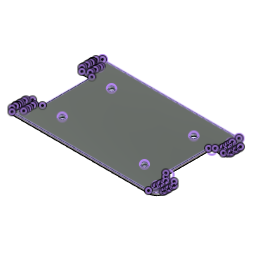
PCB Base (Autodesk Fusion 360 design; units mm, degrees)
Autodesk Fusion 360 part; units mm, degrees
note: some values were not read from the file. Set by a fixed rule: which sketch regions a step uses.
sketch "Sketch1" plane through (0, 0, 0) normal (0, 0, 1) x (1, 0, 0)
  line L0 (45, 27.5) -> (-45, 27.5)
  line L1 (-45, 27.5) -> (-45, -27.5)
  line L2 (-45, -27.5) -> (45, -27.5)
  line L3 (45, -27.5) -> (45, 27.5)
  line L4 (45, 27.5) -> (-45, -27.5) construction
  line L5 (-45, 27.5) -> (45, -27.5) construction
  dimension "d1" = 90
  dimension "d2" = 55
  constraint horizontal L0
  constraint perpendicular L0 L1
  constraint parallel L0 L2
  constraint parallel L1 L3
  constraint coincident L4 origin
  constraint coincident L5 origin
  measures "d1" distance of L1.end L2.end
  measures "d2" distance of L0.end L1.end
extrude "Extrude1" add sketch "Sketch1" along normal blind 1.6
fillet "Fillet1" radius 5 2 edges at (45, -27.5, 0.8) (45, 27.5, 0.8)
sketch "Sketch2" plane through (0, 0, 1.6) normal (0, 0, 1) x (-1, 0, 0)
  line L0 (45, -27.5) -> (45, 27.5)
  line L1 (45, 27.5) -> (-40, 27.5)
  arc A0 (-40, 27.5) -> (-45, 22.5) centre (-40, 22.5) ccw
  line L2 (-45, 22.5) -> (-45, -22.5)
  arc A1 (-45, -22.5) -> (-40, -27.5) centre (-40, -22.5) ccw
  line L3 (-40, -27.5) -> (45, -27.5)
  line L4 (25, 15) -> (-25, 15) construction
  line L5 (-25, 15) -> (-25, -15)
  line L6 (-25, -15) -> (25, -15) construction
  line L7 (25, -15) -> (25, 15)
  line L8 (25, 15) -> (-25, -15) construction
  line L9 (-25, 15) -> (25, -15) construction
  circle A2 centre (25, -15) radius 2
  circle A3 centre (25, 15) radius 1.8001
  circle A4 centre (-25, 15) radius 1.8646
  circle A5 centre (-25, -15) radius 2
  dimension "d10" = 50
  dimension "d11" = 30
  constraint horizontal L4
  constraint perpendicular L4 L5
  constraint parallel L4 L6
  constraint parallel L5 L7
  constraint coincident L8 origin
  constraint coincident L9 origin
  constraint coincident L6.end L7.start
  constraint coincident L4.start L7.end
  constraint coincident L4.end L5.start
  constraint coincident L5.end L6.start
  measures "d10" distance of L5.end L6.end
  measures "d11" distance of L4.end L5.end
extrude "Extrude2" cut sketch "Sketch2" against normal blind 4 contours A2 | A3 | A4 | A5
sketch "Sketch3" plane through (0, 0, 0) normal (0, 0, -1) x (1, 0, 0)
  circle A0 centre (25, -15) radius 2
  circle A1 centre (25, 15) radius 1.8646
  circle A2 centre (-25, -15) radius 2
  circle A3 centre (-25, 15) radius 1.8001
  line L0 (-45, -27.5) -> (40, -27.5)
  arc A4 (40, -27.5) -> (45, -22.5) centre (40, -22.5) ccw
  line L1 (45, -22.5) -> (45, 22.5)
  arc A5 (45, 22.5) -> (40, 27.5) centre (40, 22.5) ccw
  line L2 (40, 27.5) -> (-45, 27.5)
  line L3 (-45, 27.5) -> (-45, -27.5)
  line L4 (-45, 15) -> (-37, 15)
  line L5 (-37, 15) -> (-37, -15)
  line L6 (-37, -15) -> (-45, -15)
  line L7 (-45, -15) -> (-45, 15)
  constraint horizontal L4
  constraint vertical L5
  constraint horizontal L6
  constraint vertical L7
extrude "Extrude3" cut sketch "Sketch3" against normal blind 3 contours L3 L4 L5 L6 L7
sketch "Sketch4" plane through (0, 0, 0) normal (0, 0, -1) x (1, 0, 0)
  line L0 (-37, -15) -> (-45, -15)
  line L1 (-45, -27.5) -> (40, -27.5)
  arc A0 (40, -27.5) -> (45, -22.5) centre (40, -22.5) ccw
  line L2 (45, -22.5) -> (45, 22.5)
  arc A1 (45, 22.5) -> (40, 27.5) centre (40, 22.5) ccw
  line L3 (40, 27.5) -> (-45, 27.5)
  line L4 (-45, 15) -> (-37, 15)
  line L5 (-37, 15) -> (-37, -15)
  circle A2 centre (25, -15) radius 2
  circle A3 centre (25, 15) radius 1.8646
  circle A4 centre (-25, -15) radius 2
  circle A5 centre (-25, 15) radius 1.8001
  line L6 (45, 15) -> (36, 15)
  line L7 (36, 15) -> (36, -15)
  line L8 (36, -15) -> (45, -15)
  line L9 (45, -15) -> (45, 15)
  line L10 (-45, -15) -> (-45, -27.5)
  line L11 (-45, 27.5) -> (-45, 15)
  constraint horizontal L6
  constraint vertical L7
  constraint horizontal L8
  constraint vertical L9
  constraint coincident L2 L6.start
extrude "Extrude4" cut sketch "Sketch4" against normal blind 6 contours L2 L6 L7 L8 L9
sketch "Sketch5" plane through (0, 0, 1.6) normal (0, 0, 1) x (-1, 0, 0)
  circle A0 centre (25, 15) radius 1.8001
  circle A1 centre (25, -15) radius 2
  circle A2 centre (-25, 15) radius 1.8646
  circle A3 centre (-25, -15) radius 2
  line L0 (45, -15) -> (37, -15)
  line L1 (37, -15) -> (37, 15)
  line L2 (37, 15) -> (45, 15)
  line L3 (45, 27.5) -> (-40, 27.5)
  arc A4 (-40, 27.5) -> (-45, 22.5) centre (-40, 22.5) ccw
  line L4 (-45, -15) -> (-45, -22.5)
  line L5 (-45, 15) -> (-36, 15)
  line L6 (-36, 15) -> (-36, -15)
  line L7 (-36, -15) -> (-45, -15)
  arc A5 (-45, -22.5) -> (-40, -27.5) centre (-40, -22.5) ccw
  line L8 (-40, -27.5) -> (45, -27.5)
  line L9 (-44.8978, -23.5058) -> (-39.8978, -23.5058)
  line L10 (-39.8978, -23.5058) -> (-39.8978, -22.5058)
  line L11 (-39.8978, -22.5058) -> (-45, -22.5)
  line L12 (-45, -21) -> (-40, -21)
  line L13 (-40, -21) -> (-40, -20)
  line L14 (-40, -20) -> (-45, -20)
  line L15 (-45, -18) -> (-40, -18)
  line L16 (-40, -18) -> (-40, -17)
  line L17 (-40, -17) -> (-45, -17)
  line L18 (45, -27.5) -> (45, -15)
  line L19 (45, 15) -> (45, 27.5)
  line L20 (-45, 22.5) -> (-45, 15)
  dimension "d20" = 5
  dimension "d21" = 1
  dimension "d22" = 1
  dimension "d23" = 1
  constraint coincident A5 L9.start
  constraint horizontal L9
  constraint perpendicular L9 L10
  constraint coincident L4.end A5.start
  constraint perpendicular L12 L13
  constraint perpendicular L15 L16
  measures "d20" distance of L9.start L9.end
  measures "d21" distance of L9.end L10.end
  measures "d22" distance of L12.end L13.end
  measures "d23" distance of L15.end L16.end
extrude "Extrude5" cut sketch "Sketch5" against normal blind 3 contours A5 L9 L10 L11 | L4 L12 L13 L14 | L4 L15 L16 L17
mirror "Mirror1" about plane through (0, 0, 0) normal (0, 1, 0) of "Extrude5"
sketch "Sketch6" plane through (0, 0, 1.6) normal (0, 0, 1) x (-1, 0, 0)
  circle A0 centre (-25, -15) radius 2
  circle A1 centre (-25, 15) radius 1.8646
  circle A2 centre (25, -15) radius 2
  circle A3 centre (25, 15) radius 1.8001
  line L0 (-44.8978, 23.5058) -> (-39.8978, 23.5058)
  line L1 (-39.8978, 23.5058) -> (-39.8978, 22.5058)
  line L2 (-39.8978, 22.5058) -> (-45, 22.5)
  line L3 (-45, 22.5) -> (-45, 21)
  line L4 (-45, 21) -> (-40, 21)
  line L5 (-40, 21) -> (-40, 20)
  line L6 (-40, 20) -> (-45, 20)
  line L7 (-45, 20) -> (-45, 18)
  line L8 (-45, 18) -> (-40, 18)
  line L9 (-40, 18) -> (-40, 17)
  line L10 (-40, 17) -> (-45, 17)
  line L11 (-45, 15) -> (-36, 15)
  line L12 (-36, 15) -> (-36, -15)
  line L13 (-36, -15) -> (-45, -15)
  line L14 (-45, -17) -> (-40, -17)
  line L15 (-40, -17) -> (-40, -18)
  line L16 (-40, -18) -> (-45, -18)
  line L17 (-45, -18) -> (-45, -20)
  line L18 (-45, -20) -> (-40, -20)
  line L19 (-40, -20) -> (-40, -21)
  line L20 (-40, -21) -> (-45, -21)
  line L21 (-45, -21) -> (-45, -22.5)
  line L22 (-45, -22.5) -> (-39.8978, -22.5058)
  line L23 (-39.8978, -22.5058) -> (-39.8978, -23.5058)
  line L24 (-39.8978, -23.5058) -> (-44.8978, -23.5058)
  arc A4 (-44.8978, -23.5058) -> (-40, -27.5) centre (-40, -22.5) ccw
  line L25 (-40, -27.5) -> (45, -27.5)
  line L26 (45, -15) -> (37, -15)
  line L27 (37, -15) -> (37, 15)
  line L28 (37, 15) -> (45, 15)
  line L29 (45, 27.5) -> (-40, 27.5)
  arc A5 (-40, 27.5) -> (-44.8978, 23.5058) centre (-40, 22.5) ccw
  line L30 (45, -27.5) -> (45, -15)
  line L31 (45, 15) -> (45, 27.5)
  line L32 (-45, 17) -> (-45, 15)
  line L33 (-45, -15) -> (-45, -17)
mirror "Mirror2" about plane through (0, 0, 0) normal (1, 0, 0) of "Extrude5"
mirror "Mirror3" about plane through (0, 0, 0) normal (1, 0, 0) of "Mirror1"
sketch "Sketch7" plane through (-45, 0, 0) normal (-1, 0, 0) x (0, -1, 0)
  line L0 (22.5, 1.6) -> (22.5, 0)
  line L1 (22.5, 0) -> (27.5, 0)
  line L2 (27.5, 0) -> (27.5, 1.6)
  line L3 (27.5, 1.6) -> (22.5, 1.6)
  line L4 (22.5, 1.6) -> (23.5, 1.6)
  line L5 (23.5, 1.6) -> (23.5, 0)
  line L6 (23.5, 0) -> (22.5, 0)
  line L7 (22.5, 0) -> (22.5, 1.6)
  constraint horizontal L4
  constraint vertical L5
  constraint horizontal L6
  constraint vertical L7
  constraint coincident L1 L5.end
  constraint coincident L0.start L3.end
extrude "Extrude6" cut sketch "Sketch7" against normal blind 0.5 contours L0 L1 L3 L4 L5 L6 L7
sketch "Sketch8" plane through (-45, 0, 0) normal (-1, 0, 0) x (0, -1, 0)
  line L0 (-22.5, 0) -> (-22.5, 1.6)
  line L1 (-22.5, 1.6) -> (-27.5, 1.6)
  line L2 (-27.5, 1.6) -> (-27.5, 0)
  line L3 (-27.5, 0) -> (-22.5, 0)
  line L4 (-22.5, 1.6) -> (-23.5, 1.6)
  line L5 (-23.5, 1.6) -> (-23.5, 0)
  line L6 (-23.5, 0) -> (-22.5, 0)
  line L7 (-22.5, 0) -> (-22.5, 1.6)
  constraint horizontal L4
  constraint vertical L5
  constraint horizontal L6
  constraint vertical L7
  constraint coincident L3 L5.end
  constraint coincident L0.end L1.start
extrude "Extrude7" cut sketch "Sketch8" against normal blind 0.5 contours L0 L1 L3 L4 L5 L6 L7
fillet "Fillet4" radius 2 2 edges at (-45, 27.5, 0.8) (-45, 15, 0.8)
fillet "Fillet5" radius 2 2 edges at (-45, -15, 0.8) (-45, -27.5, 0.8)
fillet "Fillet6" radius 2 4 edges at (45, -15, 0.8) (36, -15, 0.8) (45, 15, 0.8) (36, 15, 0.8)
sketch "Sketch9" plane through (0, 0, 0) normal (0, 0, -1) x (1, 0, 0)
  arc A0 (45, -17) -> (43, -15) centre (43, -17) ccw
  line L0 (43, -15) -> (38, -15)
  arc A1 (36, -13) -> (38, -15) centre (38, -13) ccw
  line L1 (36, -13) -> (36, 13)
  arc A2 (38, 15) -> (36, 13) centre (38, 13) ccw
  line L2 (38, 15) -> (43, 15)
  arc A3 (43, 15) -> (45, 17) centre (43, 17) ccw
  line L3 (45, 17) -> (40, 17)
  line L4 (40, 17) -> (40, 18)
  line L5 (40, 18) -> (45, 18)
  line L6 (45, 18) -> (45, 20)
  line L7 (45, 20) -> (40, 20)
  line L8 (40, 20) -> (40, 21)
  line L9 (40, 21) -> (45, 21)
  line L10 (45, 21) -> (45, 22.5)
  line L11 (45, 22.5) -> (39.8978, 22.5058)
  line L12 (39.8978, 22.5058) -> (39.8978, 23.5058)
  line L13 (39.8978, 23.5058) -> (44.8978, 23.5058)
  arc A4 (44.8978, 23.5058) -> (40, 27.5) centre (40, 22.5) ccw
  line L14 (40, 27.5) -> (-43, 27.5)
  arc A5 (-43, 27.5) -> (-45, 25.5) centre (-43, 25.5) ccw
  line L15 (-45, 25.5) -> (-45, 23.5)
  line L16 (-45, 23.5) -> (-44.899, 23.5)
  arc A6 (-44.8978, 23.5058) -> (-44.899, 23.5) centre (-40, 22.5) ccw
  line L17 (-44.8978, 23.5058) -> (-39.8978, 23.5058)
  line L18 (-39.8978, 23.5058) -> (-39.8978, 22.5058)
  line L19 (-39.8978, 22.5058) -> (-44.5, 22.5006)
  line L20 (-44.5, 22.5006) -> (-44.5, 22.5)
  line L21 (-44.5, 22.5) -> (-45, 22.5)
  line L22 (-45, 22.5) -> (-45, 21)
  line L23 (-45, 21) -> (-40, 21)
  line L24 (-40, 21) -> (-40, 20)
  line L25 (-40, 20) -> (-45, 20)
  line L26 (-45, 20) -> (-45, 18)
  line L27 (-45, 18) -> (-40, 18)
  line L28 (-40, 18) -> (-40, 17)
  line L29 (-40, 17) -> (-45, 17)
  arc A7 (-45, 17) -> (-43, 15) centre (-43, 17) ccw
  line L30 (-43, 15) -> (-37, 15)
  line L31 (-37, 15) -> (-37, -15)
  line L32 (-37, -15) -> (-43, -15)
  arc A8 (-43, -15) -> (-45, -17) centre (-43, -17) ccw
  line L33 (-45, -17) -> (-40, -17)
  line L34 (-40, -17) -> (-40, -18)
  line L35 (-40, -18) -> (-45, -18)
  line L36 (-45, -18) -> (-45, -20)
  line L37 (-45, -20) -> (-40, -20)
  line L38 (-40, -20) -> (-40, -21)
  line L39 (-40, -21) -> (-45, -21)
  line L40 (-45, -21) -> (-45, -22.5)
  line L41 (-45, -22.5) -> (-44.5, -22.5)
  line L42 (-44.5, -22.5) -> (-44.5, -22.5006)
  line L43 (-44.5, -22.5006) -> (-39.8978, -22.5058)
  line L44 (-39.8978, -22.5058) -> (-39.8978, -23.5058)
  line L45 (-39.8978, -23.5058) -> (-44.8978, -23.5058)
  arc A9 (-44.899, -23.5) -> (-44.8978, -23.5058) centre (-40, -22.5) ccw
  line L46 (-44.899, -23.5) -> (-45, -23.5)
  line L47 (-45, -23.5) -> (-45, -25.5)
  arc A10 (-45, -25.5) -> (-43, -27.5) centre (-43, -25.5) ccw
  line L48 (-43, -27.5) -> (40, -27.5)
  arc A11 (40, -27.5) -> (44.8978, -23.5058) centre (40, -22.5) ccw
  line L49 (44.8978, -23.5058) -> (39.8978, -23.5058)
  line L50 (39.8978, -23.5058) -> (39.8978, -22.5058)
  line L51 (39.8978, -22.5058) -> (45, -22.5)
  line L52 (45, -22.5) -> (45, -21)
  line L53 (45, -21) -> (40, -21)
  line L54 (40, -21) -> (40, -20)
  line L55 (40, -20) -> (45, -20)
  line L56 (45, -20) -> (45, -18)
  line L57 (45, -18) -> (40, -18)
  line L58 (40, -18) -> (40, -17)
  line L59 (40, -17) -> (45, -17)
  circle A12 centre (25, -15) radius 2
  circle A13 centre (25, 15) radius 1.8646
  circle A14 centre (-25, -15) radius 2
  circle A15 centre (-25, 15) radius 1.8001
sketch "Sketch10" plane through (0, 0, 1.6) normal (0, 0, 1) x (-1, 0, 0)
  circle A0 centre (25, 15) radius 1.8001
  circle A1 centre (25, -15) radius 2
  circle A2 centre (-25, 15) radius 1.8646
  circle A3 centre (-25, -15) radius 2
  arc A4 (-43, -15) -> (-45, -17) centre (-43, -17) ccw
  line L0 (-45, -17) -> (-40, -17)
  line L1 (-40, -17) -> (-40, -18)
  line L2 (-40, -18) -> (-45, -18)
  line L3 (-45, -18) -> (-45, -20)
  line L4 (-45, -20) -> (-40, -20)
  line L5 (-40, -20) -> (-40, -21)
  line L6 (-40, -21) -> (-45, -21)
  line L7 (-45, -21) -> (-45, -22.5)
  line L8 (-45, -22.5) -> (-39.8978, -22.5058)
  line L9 (-39.8978, -22.5058) -> (-39.8978, -23.5058)
  line L10 (-39.8978, -23.5058) -> (-44.8978, -23.5058)
  arc A5 (-44.8978, -23.5058) -> (-40, -27.5) centre (-40, -22.5) ccw
  line L11 (-40, -27.5) -> (43, -27.5)
  arc A6 (43, -27.5) -> (45, -25.5) centre (43, -25.5) ccw
  line L12 (45, -25.5) -> (45, -23.5)
  line L13 (45, -23.5) -> (44.899, -23.5)
  arc A7 (44.8978, -23.5058) -> (44.899, -23.5) centre (40, -22.5) ccw
  line L14 (44.8978, -23.5058) -> (39.8978, -23.5058)
  line L15 (39.8978, -23.5058) -> (39.8978, -22.5058)
  line L16 (39.8978, -22.5058) -> (44.5, -22.5006)
  line L17 (44.5, -22.5006) -> (44.5, -22.5)
  line L18 (44.5, -22.5) -> (45, -22.5)
  line L19 (45, -22.5) -> (45, -21)
  line L20 (45, -21) -> (40, -21)
  line L21 (40, -21) -> (40, -20)
  line L22 (40, -20) -> (45, -20)
  line L23 (45, -20) -> (45, -18)
  line L24 (45, -18) -> (40, -18)
  line L25 (40, -18) -> (40, -17)
  line L26 (40, -17) -> (45, -17)
  arc A8 (45, -17) -> (43, -15) centre (43, -17) ccw
  line L27 (43, -15) -> (37, -15)
  line L28 (37, -15) -> (37, 15)
  line L29 (37, 15) -> (43, 15)
  arc A9 (43, 15) -> (45, 17) centre (43, 17) ccw
  line L30 (45, 17) -> (40, 17)
  line L31 (40, 17) -> (40, 18)
  line L32 (40, 18) -> (45, 18)
  line L33 (45, 18) -> (45, 20)
  line L34 (45, 20) -> (40, 20)
  line L35 (40, 20) -> (40, 21)
  line L36 (40, 21) -> (45, 21)
  line L37 (45, 21) -> (45, 22.5)
  line L38 (45, 22.5) -> (44.5, 22.5)
  line L39 (44.5, 22.5) -> (44.5, 22.5006)
  line L40 (44.5, 22.5006) -> (39.8978, 22.5058)
  line L41 (39.8978, 22.5058) -> (39.8978, 23.5058)
  line L42 (39.8978, 23.5058) -> (44.8978, 23.5058)
  arc A10 (44.899, 23.5) -> (44.8978, 23.5058) centre (40, 22.5) ccw
  line L43 (44.899, 23.5) -> (45, 23.5)
  line L44 (45, 23.5) -> (45, 25.5)
  arc A11 (45, 25.5) -> (43, 27.5) centre (43, 25.5) ccw
  line L45 (43, 27.5) -> (-40, 27.5)
  arc A12 (-40, 27.5) -> (-44.8978, 23.5058) centre (-40, 22.5) ccw
  line L46 (-44.8978, 23.5058) -> (-39.8978, 23.5058)
  line L47 (-39.8978, 23.5058) -> (-39.8978, 22.5058)
  line L48 (-39.8978, 22.5058) -> (-45, 22.5)
  line L49 (-45, 22.5) -> (-45, 21)
  line L50 (-45, 21) -> (-40, 21)
  line L51 (-40, 21) -> (-40, 20)
  line L52 (-40, 20) -> (-45, 20)
  line L53 (-45, 20) -> (-45, 18)
  line L54 (-45, 18) -> (-40, 18)
  line L55 (-40, 18) -> (-40, 17)
  line L56 (-40, 17) -> (-45, 17)
  arc A13 (-45, 17) -> (-43, 15) centre (-43, 17) ccw
  line L57 (-43, 15) -> (-38, 15)
  arc A14 (-36, 13) -> (-38, 15) centre (-38, 13) ccw
  line L58 (-36, 13) -> (-36, -13)
  arc A15 (-38, -15) -> (-36, -13) centre (-38, -13) ccw
  line L59 (-38, -15) -> (-43, -15)
  line L60 (43, -27.5) -> (-40, -27.5)
